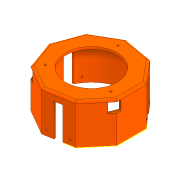
# Autodesk Inventor part: Delts Robot Casing
Saved by Autodesk Inventor 2020 (Build 240168000, 168)
## iProperties
Created: 2021-03-07
Part Number: Delts Robot Casing
Material: Generic
Document SubType Name: Modeling
Designer: Coy
Density: 1 g/cm^3
Appearance: Default(1)
Author: Coy
Autodesk Inventor part; units mm, degrees
ref_plane "YZ Plane" through (0, 0, 0) normal (1, 0, 0) x (0, 1, 0)
ref_plane "XZ Plane" through (0, 0, 0) normal (0, 1, 0) x (-1, 0, 0)
ref_plane "XY Plane" through (0, 0, 0) normal (0, 0, 1) x (1, 0, 0)
sketch "Sketch1" plane through (0, 0, 0) normal (0, 1, 0) x (-1, 0, 0)
  line L0 (-78.0093, 17.2136) -> (-78.0093, 27.2133) construction
  line L1 (-78.0093, 27.2133) -> (-68.0093, 27.2133) construction
  line L2 (-68.0093, 27.2133) -> (-68.0093, 17.2136) construction
  line L3 (-68.0093, 17.2136) -> (-47.6421, 17.2136) construction
  line L4 (-47.6421, 17.2136) -> (-47.6421, 7.2136) construction
  line L5 (-82.2526, 7.2136) -> (-20.6847, 7.2136) construction
  line L6 (-20.6847, 7.2136) -> (-20.6847, -6.7867) construction
  line L7 (-82.2527, -6.7867) -> (-5, -6.7867) construction
  line L8 (-5, -6.7867) -> (-5, -6.879) construction
  line L9 (-5, -6.879) -> (-22.1607, -16.7867) construction
  line L10 (-22.1607, -16.7867) -> (-80.7806, -16.7867) construction
  arc A0 (-80.7806, -16.7867) -> (25.6679, -78.2448) centre (0, 0.2133) ccw construction
  line L11 (25.6679, -78.2448) -> (24.2822, -75.8448) construction
  line L12 (24.2822, -75.8448) -> (15.622, -80.8448) construction
  line L13 (15.622, -80.8448) -> (10.622, -72.1845) construction
  line L14 (10.622, -72.1845) -> (19.2822, -67.1845) construction
  line L15 (19.2822, -67.1845) -> (9.0986, -49.546) construction
  line L16 (9.0986, -49.546) -> (17.7589, -44.546) construction
  line L17 (35.0642, -74.5196) -> (4.3725, -21.3602) construction
  line L18 (4.3725, -21.3602) -> (16.4969, -14.3602) construction
  line L19 (47.1885, -67.5196) -> (8.5622, -0.6169) construction
  line L20 (8.5622, -0.6169) -> (8.6421, -0.5707) construction
  line L21 (8.6421, -0.5707) -> (25.8028, -10.4785) construction
  line L22 (25.8028, -10.4785) -> (55.1127, -61.2448) construction
  line L23 (55.1127, 61.6713) -> (53.7271, 59.2713) construction
  line L24 (53.7271, 59.2713) -> (60.2914, 55.4814) construction
  line L25 (60.2914, 55.4814) -> (56.294, 47.8224) construction
  line L26 (56.294, 47.8224) -> (47.4289, 52.4494) construction
  line L27 (47.4289, 52.4494) -> (38.0051, 34.3935) construction
  line L28 (38.0051, 34.3935) -> (29.1399, 39.0204) construction
  line L29 (45.0044, 69.4166) -> (16.5814, 14.9585) construction
  line L30 (16.5814, 14.9585) -> (4.1702, 21.4362) construction
  line L31 (4.1702, 21.4362) -> (-3.5622, 8.0434) construction
  line L32 (-3.5622, 8.0434) -> (-3.6421, 8.0895) construction
  line L33 (-3.6421, 8.0895) -> (-3.6421, 27.905) construction
  line L34 (-3.6421, 27.905) -> (25.6679, 78.6713) construction
  line L35 (-80.7805, 17.2136) -> (-78.0093, 17.2136) construction
  line L36 (4.1702, 21.4362) -> (35.0642, 74.9462) construction
  arc A1 (25.6679, -78.2448) -> (35.0642, -74.5196) centre (0, 0.2133) ccw construction
  arc A2 (47.1885, -67.5196) -> (45.0044, 69.4166) centre (0, 0.2133) ccw construction
  arc A3 (35.0642, 74.9462) -> (-82.2526, 7.2136) centre (0, 0.2133) ccw construction
  arc A4 (-82.2527, -6.7867) -> (-80.7806, -16.7867) centre (0, 0.2133) ccw construction
  circle A5 centre (0, 0.2133) radius 83.05
  line L37 (-86.05, 31.5329) -> (-45.7862, 79.5174)
  line L38 (-45.7862, 79.5174) -> (15.9014, 90.3946)
  line L39 (15.9014, 90.3946) -> (70.1486, 59.0749)
  line L40 (70.1486, 59.0749) -> (91.5725, 0.2133)
  line L41 (91.5725, 0.2133) -> (70.1486, -58.6484)
  line L42 (70.1486, -58.6484) -> (15.9014, -89.968)
  line L43 (15.9014, -89.968) -> (-45.7862, -79.0908)
  line L44 (-45.7862, -79.0908) -> (-86.05, -31.1064)
  line L45 (-86.05, -31.1064) -> (-86.05, 31.5329)
  point P0 (0, 0)
  point P1 (0, 0)
  dimension "d0" = 166.1
  dimension "d1" = 3
  constraints: 92 end point, 14 point on circle, 6 centre point, 5 point on line, 2 coincident, 1 collinear, 19 other
  measures "d0" diameter of A5
  measures "d1" distance edge to line of A5 L45
extrude "Extrusion1" add sketch "Sketch1" along normal blind 60
sketch "Sketch2" plane through (-91.5725, 0, 0.2133) normal (-0.9396926, 0, -0.3420201) x (-0.3420201, 0, 0.9396926)
  line L0 (-62.6393, 60) -> (0, 60) projected
  line L1 (-31.3196, 60) -> (-31.3196, 0) construction
  line L2 (-62.6393, 0) -> (0, 0) projected
  line L3 (-23.8125, 60) -> (-23.8125, 0)
  line L4 (-39.6875, 60) -> (-39.6875, 0)
  point P0 (-31.52, 0)
  point P1 (-39.6875, 0)
  point P2 (-23.8125, 0)
  dimension "d4" = 7.5071
  dimension "d5" = 8.3679
  constraints: 6 end point, 2 midpoint, 2 parallel, 1 perpendicular
  measures "d4" distance between parallel lines of L1 L3
  measures "d5" distance between parallel lines of L1 L4
extrude "Extrusion2" cut sketch "Sketch2" against normal blind 60
sketch "Sketch3" plane through (-70.1486, 0, -58.6484) normal (-0.9396926, 0, -0.3420201) x (-0.3420201, 0, 0.9396926)
  line L0 (0, 60) -> (22.9518, 60) construction
  line L1 (9.3198, 60) -> (9.3198, 0) construction
  line L2 (22.9518, 0) -> (22.9518, 60) construction
  circle A0 centre (9.3198, 11) radius 1.625
  line L3 (0, 0) -> (22.9518, 0) projected
  point P0 (31.1192, 0)
  dimension "d8" = 13.632
  dimension "d9" = 3.25
  dimension "d10" = 11
  constraints: 2 end point, 2 point on line, 1 centre point, 1 vertical
  measures "d8" distance between parallel lines of L2 L1
  measures "d9" diameter of A0
  measures "d10" distance from line of L3 A0.centre
extrude "Extrusion3" cut sketch "Sketch3" against normal blind 60
sketch "Sketch4" plane through (45.7862, 0, 79.5174) normal (0.1736482, 0, 0.9848078) x (0.9848078, 0, -0.1736482)
  line L0 (-62.6393, 60) -> (0, 60) projected
  line L1 (-31.3196, 60) -> (-31.3196, 0) construction
  line L2 (-62.6393, 0) -> (0, 0) projected
  line L3 (-23.8125, 60) -> (-23.8125, 0)
  line L4 (-39.6875, 60) -> (-39.6875, 0)
  point P0 (-31.2826, 0)
  point P1 (-98.6931, 60)
  point P2 (-106.7022, 60)
  point P3 (-31.3196, 0)
  point P4 (-39.6875, 60)
  point P5 (-39.6875, 0)
  point P6 (-23.8125, 0)
  point P7 (-23.8125, 60)
  dimension "d13" = 7.5071
  dimension "d14" = 8.3679
  constraints: 6 end point, 2 midpoint, 2 parallel, 1 vertical
  measures "d13" distance between parallel lines of L1 L3
  measures "d14" distance between parallel lines of L1 L4
extrude "Extrusion4" cut sketch "Sketch4" against normal blind 60
sketch "Sketch5" plane through (-15.9014, 0, 90.3946) normal (0.1736482, 0, 0.9848078) x (0.9848078, 0, -0.1736482)
  line L0 (31.3196, 60) -> (-27.542, 60) construction
  line L1 (9.3198, 60) -> (9.3198, 0) construction
  line L2 (22.9518, 0) -> (22.9518, 60) construction
  circle A0 centre (9.3198, 11) radius 1.625
  line L3 (0, 0) -> (22.9518, 0) projected
  point P0 (31.3567, 0)
  dimension "d17" = 13.632
  dimension "d18" = 3.25
  dimension "d19" = 11
  constraints: 2 end point, 2 point on line, 1 centre point, 1 vertical
  measures "d17" distance between parallel lines of L2 L1
  measures "d18" diameter of A0
  measures "d19" distance from line of L3 A0.centre
extrude "Extrusion5" cut sketch "Sketch5" against normal blind 60
sketch "Sketch6" plane through (45.7862, 0, -79.0908) normal (0.7660444, 0, -0.6427876) x (-0.6427876, 0, -0.7660444)
  line L0 (-62.6393, 60) -> (0, 60) projected
  line L1 (-31.3196, 60) -> (-31.3196, 0) construction
  line L2 (-62.6393, 0) -> (0, 0) projected
  line L3 (-23.8125, 60) -> (-23.8125, 0)
  line L4 (-39.6875, 60) -> (-39.6875, 0)
  point P0 (-31.3196, 0)
  point P1 (-39.6875, 60)
  point P2 (-39.6875, 0)
  point P3 (-23.8125, 0)
  point P4 (-23.8125, 60)
  dimension "d22" = 7.5071
  dimension "d23" = 8.3679
  constraints: 6 end point, 2 midpoint, 2 parallel, 1 vertical
  measures "d22" distance between parallel lines of L1 L3
  measures "d23" distance between parallel lines of L1 L4
extrude "Extrusion6" cut sketch "Sketch6" against normal blind 60
sketch "Sketch7" plane through (86.05, 0, -31.1064) normal (0.7660444, 0, -0.6427876) x (-0.6427876, 0, -0.7660444)
  line L0 (-36.0538, 60) -> (99.195, 60) construction
  line L1 (33.3375, 60) -> (33.3375, 0) construction
  line L2 (-36.0538, 0) -> (99.195, 0) construction
  line L3 (-51.7304, 60) -> (22.9518, 60) construction
  line L4 (9.3198, 60) -> (9.3198, 0) construction
  line L5 (-51.7304, 0) -> (22.9518, 0) construction
  line L6 (22.9518, 0) -> (22.9518, 60) construction
  circle A0 centre (9.3198, 11) radius 1.625
  point P0 (31.483, 0)
  point P1 (-44.0629, 60)
  point P2 (-44.0629, 0)
  dimension "d26" = 13.632
  dimension "d27" = 3.25
  dimension "d28" = 11
  constraints: 5 point on line, 4 end point, 1 centre point, 1 perpendicular, 1 vertical
  measures "d26" distance between parallel lines of L6 L4
  measures "d27" diameter of A0
  measures "d28" distance from line of L2 A0.centre
extrude "Extrusion7" cut sketch "Sketch7" against normal blind 60
sketch "Sketch8" plane through (45.7862, 0, -79.0908) normal (0.7660444, 0, -0.6427876) x (-0.6427876, 0, -0.7660444)
  circle A0 centre (-53.3195, 11) radius 1.625 projected
  line L0 (-31.1563, 0) -> (-31.1563, 65.0875) construction
  circle A1 centre (-8.993, 11) radius 1.625
  constraints: 2 end point, 1 centre point, 1 symmetric about line, 1 vertical, 1 other
extrude "Extrusion8" cut sketch "Sketch8" against normal blind 60 contours A1
sketch "Sketch9" plane through (-70.1486, 0, -58.6484) normal (-0.9396926, 0, -0.3420201) x (-0.3420201, 0, 0.9396926)
  circle A0 centre (9.3198, 11) radius 1.625 projected
  line L0 (31.1192, 0) -> (31.1192, 73.025) construction
  circle A1 centre (52.9187, 11) radius 1.625
  constraints: 2 end point, 1 centre point, 1 symmetric about line, 1 vertical, 1 other
extrude "Extrusion9" cut sketch "Sketch9" against normal blind 60 contours A1
sketch "Sketch10" plane through (-15.9014, 0, 90.3946) normal (0.1736482, 0, 0.9848078) x (0.9848078, 0, -0.1736482)
  circle A0 centre (9.3198, 11) radius 1.625 projected
  line L0 (90.1813, 0) -> (31.3196, 0) construction
  line L1 (31.3196, 0) -> (31.3196, 21.1493) construction
  line L2 (31.3196, 0) -> (31.3196, 60) construction
  circle A1 centre (53.3195, 11) radius 1.625
  point P0 (31.3567, 0)
  constraints: 2 end point, 1 centre point, 1 point on line, 1 symmetric about line, 1 other
extrude "Extrusion10" cut sketch "Sketch10" against normal blind 60 contours A1
sketch "Sketch11" plane through (0, 60, 0) normal (0, 1, 0) x (1, 0, 0)
  line L0 (-0.2166, -13.8885) -> (-13.7151, 2.1984) construction
  line L1 (-13.7151, 2.1984) -> (6.9658, 5.845) construction
  line L2 (6.9658, 5.845) -> (-0.2166, -13.8885) construction
  line L3 (86.05, 31.1064) -> (71.2969, 48.6885) construction
  line L4 (22.3355, -83.6524) -> (45.7862, -79.5174) construction
  line L5 (86.05, 31.1064) -> (45.7862, -79.5174) construction
  line L6 (-70.1486, -59.0749) -> (-15.9014, -90.3946) construction
  line L7 (-83.4281, 22.1632) -> (-91.5725, -0.2133) construction
  line L8 (-15.9014, -90.3946) -> (-91.5725, -0.2133) construction
  line L9 (45.7862, 79.0908) -> (-15.9014, 89.968) construction
  line L10 (-70.1486, 58.6484) -> (-77.9986, 37.0808) construction
  line L11 (45.7862, 79.0908) -> (-70.1486, 58.6484) construction
  line L12 (6.9658, 5.845) -> (-6.9658, -5.845) construction
  line L13 (-0.2166, -13.8885) -> (6.9658, 5.845) construction
  line L14 (6.9658, 5.845) -> (133.0894, -40.0602)
  line L15 (133.0894, -40.0602) -> (125.9069, -59.7937) construction
  line L16 (125.9069, -59.7937) -> (-0.2166, -13.8885)
  line L17 (-13.7151, 2.1984) -> (-0.2166, -13.8885) construction
  line L18 (-0.2166, -13.8885) -> (-97.6692, -95.661)
  line L19 (-97.6692, -95.661) -> (-111.1677, -79.574) construction
  line L20 (-111.1677, -79.574) -> (-13.7151, 2.1984)
  line L21 (-13.7151, 2.1984) -> (6.9658, 5.845) construction
  line L22 (6.9658, 5.845) -> (-16.1009, 136.6631)
  line L23 (-16.1009, 136.6631) -> (-36.7819, 133.0165) construction
  line L24 (-36.7819, 133.0165) -> (-13.7151, 2.1984)
  line L25 (58.534, 58.7025) -> (61.0926, 60.8494) projected
  line L26 (61.0926, 60.8494) -> (45.7862, 79.0908) projected
  line L27 (45.7862, 79.0908) -> (-15.9014, 89.968) projected
  line L28 (-15.9014, 89.968) -> (-70.1486, 58.6484) projected
  line L29 (-70.1486, 58.6484) -> (-77.9986, 37.0808) projected
  line L30 (-77.9986, 37.0808) -> (-74.7823, 35.9102) projected
  arc A0 (58.534, 58.7025) -> (-74.7823, 35.9102) centre (0, -0.2133) ccw projected
  line L31 (6.7017, -86.409) -> (6.1074, -83.0384) projected
  arc A1 (-80.2896, 21.0208) -> (6.1074, -83.0384) centre (0, -0.2133) ccw projected
  line L32 (-80.2896, 21.0208) -> (-83.4281, 22.1632) projected
  line L33 (-83.4281, 22.1632) -> (-91.5725, -0.2133) projected
  line L34 (-91.5725, -0.2133) -> (-70.1486, -59.0749) projected
  line L35 (-70.1486, -59.0749) -> (-15.9014, -90.3946) projected
  line L36 (-15.9014, -90.3946) -> (6.7017, -86.409) projected
  line L37 (71.2969, 48.6885) -> (68.675, 46.4884) projected
  arc A2 (21.7555, -80.3631) -> (68.675, 46.4884) centre (0, -0.2133) ccw projected
  line L38 (21.7555, -80.3631) -> (22.3355, -83.6524) projected
  line L39 (22.3355, -83.6524) -> (45.7862, -79.5174) projected
  line L40 (45.7862, -79.5174) -> (86.05, -31.5329) projected
  line L41 (86.05, -31.5329) -> (86.05, 31.1064) projected
  line L42 (86.05, 31.1064) -> (71.2969, 48.6885) projected
  arc A3 (-80.2896, 21.0208) -> (6.1074, -83.0384) centre (0, -0.2133) ccw projected
  circle A4 centre (0, -0.2133) radius 83.05
  line L43 (-77.9986, 37.0808) -> (-74.7823, 35.9102) projected
  line L44 (-77.9986, 37.0808) -> (-83.4281, 22.1632)
  line L45 (-15.9014, -90.3946) -> (6.7017, -86.409) projected
  line L46 (6.7017, -86.409) -> (22.3355, -83.6524)
  line L47 (61.0926, 60.8494) -> (45.7862, 79.0908) projected
  line L48 (71.2969, 48.6885) -> (61.0926, 60.8494)
  point P0 (0, 0)
  point P1 (0, 0)
  point P2 (77.2091, -42.0691)
  point P3 (72.6702, -40.4171)
  point P4 (21.7555, -80.3631)
  point P5 (-56.481, -61.1)
  point P6 (-60.6223, -64.5749)
  point P7 (-74.0298, -48.4116)
  point P8 (-69.9477, -44.9863)
  point P9 (-27.1304, 78.2803)
  point P10 (-27.9633, 83.0041)
  point P11 (-7.6095, 88.506)
  point P12 (-6.5641, 82.5769)
  point P13 (80.4336, -20.895)
  point P14 (86.05, -22.9392)
  dimension "d37" = 21
  dimension "d38" = 0
  dimension "d39" = 0
  constraints: 44 end point, 9 parallel, 5 collinear, 4 perpendicular, 2 midpoint, 1 coincident, 3 other
  measures "d37" distance of L0.start L0.end
  measures "d38" distance of point (0, 0) point (0, 0)
  measures "d39" distance of point (0, 0) point (0, 0)
extrude "Extrusion11" add sketch "Sketch11" along normal blind 21 contours A2 L37 L42 L41 L14 | L22 L27 L26 L25 A0 | L16 L40 L39 L38 A2 | L25 L48 L37 A4 | A0 L30 L29 L28 L24 | L38 L46 L31 A4 | A4 L32 L44 L30 | A1 L31 L36 L35 L18 | L20 L34 L33 L32 A1
sketch "Sketch13" plane through (0, 81, 0) normal (0, 1, 0) x (1, 0, 0)
  arc A0 (80.4336, -20.895) -> (-6.5641, 82.5769) centre (0, -0.2133) ccw projected
  line L0 (80.4336, -20.895) -> (86.05, -22.9392) projected
  line L1 (86.05, -22.9392) -> (86.05, 31.1064) projected
  line L2 (86.05, 31.1064) -> (45.7862, 79.0908) projected
  line L3 (45.7862, 79.0908) -> (-7.6095, 88.506) projected
  line L4 (-7.6095, 88.506) -> (-6.5641, 82.5769) projected
  line L5 (45.7862, -79.5174) -> (77.2091, -42.0691) projected
  line L6 (77.2091, -42.0691) -> (72.6702, -40.4171) projected
  arc A1 (-56.481, -61.1) -> (72.6702, -40.4171) centre (0, -0.2133) ccw projected
  line L7 (-56.481, -61.1) -> (-60.6223, -64.5749) projected
  line L8 (-60.6223, -64.5749) -> (-15.9014, -90.3946) projected
  line L9 (-15.9014, -90.3946) -> (45.7862, -79.5174) projected
  line L10 (-27.9633, 83.0041) -> (-70.1486, 58.6484) projected
  line L11 (-70.1486, 58.6484) -> (-91.5725, -0.2133) projected
  line L12 (-91.5725, -0.2133) -> (-74.0298, -48.4116) projected
  line L13 (-74.0298, -48.4116) -> (-69.9477, -44.9863) projected
  arc A2 (-27.1304, 78.2803) -> (-69.9477, -44.9863) centre (0, -0.2133) ccw projected
  line L14 (-27.1304, 78.2803) -> (-27.9633, 83.0041) projected
  line L15 (-27.9633, 83.0041) -> (-27.1304, 78.2803) projected
  arc A3 (-6.5641, 82.5769) -> (-27.1304, 78.2803) centre (0, -0.2133) ccw projected
  line L16 (-6.5641, 82.5769) -> (-7.6095, 88.506) projected
  line L17 (-7.6095, 88.506) -> (-15.9014, 89.968) projected
  line L18 (-15.9014, 89.968) -> (-27.9633, 83.0041) projected
  line L19 (-60.6223, -64.5749) -> (-56.481, -61.1) projected
  arc A4 (-69.9477, -44.9863) -> (-56.481, -61.1) centre (0, -0.2133) ccw projected
  line L20 (-69.9477, -44.9863) -> (-74.0298, -48.4116) projected
  line L21 (-74.0298, -48.4116) -> (-70.1486, -59.0749) projected
  line L22 (-70.1486, -59.0749) -> (-60.6223, -64.5749) projected
  line L23 (72.6702, -40.4171) -> (77.2091, -42.0691) projected
  line L24 (77.2091, -42.0691) -> (86.05, -31.5329) projected
  line L25 (86.05, -31.5329) -> (86.05, -22.9392) projected
  line L26 (86.05, -22.9392) -> (80.4336, -20.895) projected
  arc A5 (72.6702, -40.4171) -> (80.4336, -20.895) centre (0, -0.2133) ccw projected
  point P0 (0, 0)
extrude "Extrusion12" add sketch "Sketch13" along normal blind 5
sketch "Sketch14" plane through (0, 86, 0) normal (0, 1, 0) x (1, 0, 0)
  line L0 (86.05, -31.5329) -> (-80.8606, 29.2176) construction
  line L1 (-70.1486, 58.6484) -> (-91.5725, -0.2133) construction
  line L2 (-7.6095, 88.506) -> (-15.9014, 89.968) construction
  line L3 (-15.9014, 89.968) -> (14.9424, -84.956) construction
  line L4 (-15.9014, -90.3946) -> (45.7862, -79.5174) construction
  line L5 (-70.1486, -59.0749) -> (-15.9014, -90.3946) construction
  line L6 (-70.1486, -59.0749) -> (66.1948, 54.7689) construction
  line L7 (71.2969, 48.6885) -> (61.0926, 60.8494) construction
  circle A0 centre (0, 0) radius 69.85 construction
  circle A1 centre (-53.3689, -45.0642) radius 1.75
  circle A2 centre (65.5687, -24.0783) radius 1.75
  circle A3 centre (-12.1658, 68.7824) radius 1.75
  dimension "d45" = 139.7
  dimension "d46" = 3.5
  dimension "d47" = 3.5
  dimension "d48" = 3.5
  constraints: 6 end point, 4 centre point, 3 midpoint, 3 point on circle, 3 point on line, 1 coincident
  measures "d45" diameter of A0
  measures "d46" diameter of A1
  measures "d47" diameter of A2
  measures "d48" diameter of A3
extrude "Extrusion13" cut sketch "Sketch14" against normal through all
sketch "Sketch16" plane through (0, 86, 0) normal (0, 1, 0) x (1, 0, 0)
  circle A0 centre (0, 0) radius 55
  dimension "d84" = 110
  constraints: 1 centre point, 1 coincident
  measures "d84" diameter of A0
extrude "Extrusion15" cut sketch "Sketch16" against normal blind 25.4
sketch "Sketch17" plane through (0, 60, 0) normal (0, -1, 0) x (1, 0, 0)
  line L0 (71.2969, -48.6885) -> (68.675, -46.4884) projected
  arc A0 (58.534, -58.7025) -> (68.675, -46.4884) centre (0, 0.2133) ccw projected
  line L1 (58.534, -58.7025) -> (61.0926, -60.8494) projected
  line L2 (71.2969, -48.6885) -> (61.0926, -60.8494) projected
  line L3 (21.7555, 80.3631) -> (22.3355, 83.6524) projected
  line L4 (6.7017, 86.409) -> (22.3355, 83.6524) projected
  line L5 (6.7017, 86.409) -> (6.1074, 83.0384) projected
  arc A1 (21.7555, 80.3631) -> (6.1074, 83.0384) centre (0, 0.2133) ccw projected
  line L6 (-77.9986, -37.0808) -> (-74.7823, -35.9102) projected
  arc A2 (-80.2896, -21.0208) -> (-74.7823, -35.9102) centre (0, 0.2133) ccw projected
  line L7 (-80.2896, -21.0208) -> (-83.4281, -22.1632) projected
  line L8 (-77.9986, -37.0808) -> (-83.4281, -22.1632) projected
  point P0 (0, 0)
extrude "Extrusion16" cut sketch "Sketch17" against normal blind 10
fillet "Fillet1" radius 5 15 edges at (-49.056, 86, -70.8262) (-21.9324, 86, -86.4861) (-80.8606, 86, -29.2176) (-82.8011, 86, 24.3124) (-72.0892, 86, 53.7432) (-65.3855, 86, 61.8249) (-38.2619, 86, 77.4848) (14.9424, 86, 84.956) (81.6295, 86, 36.801) (61.4977, 86, 60.7933) (86.05, 86, -4.0836) (86.05, 86, 27.2361) (65.9181, 86, -55.0986) (-11.7555, 86, -89.237) (19.0884, 86, -83.7984)
sketch "Sketch18" plane through (0, 0, 0) normal (0, -1, 0) x (1, 0, 0)
  line L0 (68.675, -46.4884) -> (71.2969, -48.6885) projected
  line L1 (86.05, -31.1064) -> (71.2969, -48.6885) projected
  line L2 (86.05, 31.5329) -> (86.05, -31.1064) projected
  line L3 (45.7862, 79.5174) -> (86.05, 31.5329) projected
  line L4 (22.3355, 83.6524) -> (45.7862, 79.5174) projected
  line L5 (22.3355, 83.6524) -> (21.7555, 80.3631) projected
  arc A0 (68.675, -46.4884) -> (21.7555, 80.3631) centre (0, 0.2133) ccw projected
  point P0 (0, 0)
body "Solid1"
